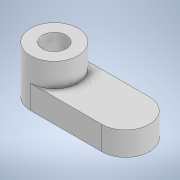
# Autodesk Inventor part: 10-18-19 D
Saved by Autodesk Inventor 2020 (Build 240168000, 168)
## iProperties
Created: 2019-10-22
Part Number: 10-18-19 D
Material: Generic
Document SubType Name: Modeling
Designer: cks4a449
Density: 1 g/cm^3
Appearance: Default
Author: cks4a449
Autodesk Inventor part; units mm, degrees
ref_plane "YZ Plane" through (0, 0, 0) normal (1, 0, 0) x (0, 1, 0)
ref_plane "XZ Plane" through (0, 0, 0) normal (0, 1, 0) x (-1, 0, 0)
ref_plane "XY Plane" through (0, 0, 0) normal (0, 0, 1) x (1, 0, 0)
sketch "Sketch1" plane through (0, 0, 0) normal (0, 1, 0) x (-1, 0, 0)
  circle A0 centre (0, 0) radius 25.4
  line L0 (-25.4, 0) -> (-25.4, -76.2)
  line L1 (25.4, -76.2) -> (25.4, 0)
  arc A1 (-25.4, -76.2) -> (25.4, -76.2) centre (0, -76.2) ccw
  circle A2 centre (0, 0) radius 12.7
  dimension "d0" = 50.8
  dimension "d1" = 76.2
  dimension "d2" = 50.8
  dimension "d3" = 25.4
  constraints: 4 end point, 4 point on circle, 3 centre point, 2 coincident, 2 tangent, 1 vertical
  measures "d0" diameter of A0
  measures "d1" distance of L0.start L0.end
  measures "d2" distance of L0.end L1.start
  measures "d3" diameter of A2
extrude "Extrusion1" add sketch "Sketch1" along normal blind 25.4 contours L1 A1 L0 A0
extrude "Extrusion2" add sketch "Sketch1" along normal blind 50.8 contours A0
body "Solid1"
